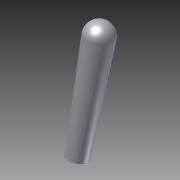
# Autodesk Inventor part: B12APtoggle
Saved by Autodesk Inventor 2011 SP1 (Build 150282100, 282)
## iProperties
Created: 2013-12-24
Part Number: B12APtoggle
Catalog Web Link: www.cadenas.de
Description: B Series - Toggle-
Vendor: NKKSWITCHES
Document SubType Name: Modeling
Designer: PARTuser1
Manufacturer: NKKSWITCHES
Density: 1 g/cm^3
Category: PARTsolutions
Company: NKKSWITCHES
Title: B12APtoggle
Author: Cadenas PARTsolutions
PSOL_IDENT_0: {$CADENAS_DATA\23d-libs\nkkswitches\toggle\b\parts\b_toggle.prj},206 {VTYP=3D},{NB=B12APtoggle},{LIN
PSOL_IDENT_1: A=B12APtoggle},{NN=B Series - Toggle},{DATE=06.03.2009 07:38:25},{GEOMDATE=05.03.2009 12:27:00},{VER
PSOL_IDENT_2: SION=},{LINEID=10},{LINESUBID=-1},{WBVAR=PLS,CRCTS,TGGLS,TRMNLS,CPS,CCLR}  {NB=B12APtoggle},{LINA=B1
PSOL_IDENT_3: 2APtoggle},{KT=DUMMY},{PN=B12AP},{SRS=B},{PLS=1},{CRCTS=2},{CRCTSALG= '2','2 - ON/NONE/ON','3','3 -
PSOL_IDENT_4: ON/OFF/ON','5','5 - ON/NONE/(ON)','R','R - (ON)/NONE/ON','8','8 - (ON)/OFF/(ON)','9','9 - ON/OFF/(ON
PSOL_IDENT_5: )','S','S - (ON)/OFF/ON' },{TGGLS=A},{TGGLSALG=  'A','A - .394\" (10.0 mm) Bat','A1','A1 - .315\" (8
PSOL_IDENT_6: .0 mm) Bat with Panel Seal Threaded Bushing  '  ,'J','J - .248\" (6.3 mm) Bat','E','E - .394\" (10.0
PSOL_IDENT_7: mm) Flatted','H','H - .248\" (6.3 mm) Flatted','K','K - Snap Top for Paddles','L','L - Locking Leve
PSOL_IDENT_8: r' },{TRMNLS=P},{TRMNLSALG= 'P','P - Straight','B','B - Straight with Bracket', 'H','H - Right Angle
PSOL_IDENT_9: with Bracket','V','V - Vertical with Bracket' ,'W','W - Straight Long' },{CPS=},{CPSALG= '','w/o Ca
PSOL_IDENT_10: p','G','G - .394\" (10.0 mm) Bat Lever Cap' },{CCLR=},{CCLR1= '', 'N/A' }
CNS_NN: B Series - Toggle
CNS_NB: B12APtoggle
CNS_NBSYN: $PN.toggle
CNS_LINA: B12APtoggle
CNS_PN: B12AP
CNS_SRS: B
CNS_PLS: 1 - SPDT
CNS_CRCTS: 2 - ON/NONE/ON
CNS_CRCTSALG: '2','2 - ON/NONE/ON','3','3 - ON/OFF/ON','5','5 - ON/NONE/(ON)','R','R - (ON)/NONE/ON','8','8 - (ON)/OFF/(ON)','9','9 - ON/OFF/(ON)','S','S - (ON)/OFF/ON'
CNS_TGGLS: A - .394" (10.0 mm) Bat
CNS_TGGLSALG: 'A','A - .394" (10.0 mm) Bat','A1','A1 - .315" (8.0 mm) Bat with Panel Seal Threaded Bushing  '  ,'J','J - .248" (6.3 mm) Bat','E','E - .394" (10.0 mm) Flatted','H','H - .248" (6.3 mm) Flatted','K','K - Snap Top for Paddles','L','L - Locking Lever'
CNS_TRMNLS: P - Straight
CNS_TRMNLSALG: 'P','P - Straight','B','B - Straight with Bracket', 'H','H - Right Angle with Bracket','V','V - Vertical with Bracket' ,'W','W - Straight Long'
CNS_CPS: w/o Cap
CNS_CPSALG: '','w/o Cap','G','G - .394" (10.0 mm) Bat Lever Cap'
CNS_CCLR: N/A
CNS_CCLR1: '', 'N/A'
SUPPLIER: NKKSWITCHES
ARTICLENO: B12APtoggle
BOMINFO: B12APtoggle
CREATOR: CADENAS GmbH
Autodesk Inventor part; units mm, degrees
sketch "Sketch_1" plane through (0, 0, 0) normal (1, 0, 0) x (0, 1, 0)
  line L0 (9.7511, -2.2512) -> (-1.016, 0.2346)
  line L1 (-1.016, 0.2346) -> (-1.016, 1.2066)
  line L2 (-1.016, 1.2066) -> (8.7803, -0.6976)
  arc A0 (9.7511, -2.2512) -> (8.7803, -0.6976) centre (8.4889, -1.9598) ccw
  line L3 (9.7511, -2.2512) -> (-1.016, 0.2346)
  constraints: 8 end point, 2 point on circle, 1 centre point
revolve "Revolution1" add sketch "Sketch_1" angle 360 about axis through (0, 9.7511, -2.2512) along (0, 0.9743701, -0.2249511)
ref_plane "1_righta_vertical_XY" through (0, 0, 0) normal (0, 0, 1) x (1, 0, 0)
ref_plane "1_righta_vertical_YZ" through (0, 0, 0) normal (1, 0, 0) x (0, 1, 0)
ref_plane "1_righta_vertical_ZX" through (0, 0, 0) normal (0, 1, 0) x (0, 0, 1)
ref_plane "1_straight_XY" through (0, 0, 0) normal (0, 1, 0) x (1, 0, 0)
ref_plane "1_straight_YZ" through (0, 0, 0) normal (1, 0, 0) x (0, 0, -1)
ref_plane "1_straight_ZX" through (0, 0, 0) normal (0, 0, -1) x (0, 1, 0)
ref_plane "right_vertical_l_XY" through (0, 0, -6.9088) normal (0, 0, 1) x (1, 0, 0)
ref_plane "right_vertical_l_YZ" through (0, 0, -6.9088) normal (1, 0, 0) x (0, 1, 0)
ref_plane "right_vertical_l_ZX" through (0, 0, -6.9088) normal (0, 1, 0) x (0, 0, 1)
ref_plane "straight_l_XY" through (0, -6.9088, 0) normal (0, 1, 0) x (1, 0, 0)
ref_plane "straight_l_YZ" through (0, -6.9088, 0) normal (1, 0, 0) x (0, 0, -1)
ref_plane "straight_l_ZX" through (0, -6.9088, 0) normal (0, 0, -1) x (0, 1, 0)
body "Solid1"
